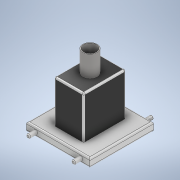
# Autodesk Inventor part: Base Prime
Saved by Autodesk Inventor 2022 (Build 260153000, 153)
## iProperties
Created: 2021-10-29
Part Number: Base Prime
Material: Aluminum 6061
Document SubType Name: Modeling
Designer: Mark Maara
Density: 2.7 g/cm^3
Appearance: Aluminum - Polished
Mass: 6995.86 g
Surface Area: 46826.5 cm^2
Volume: 2591.06 cm^3
Author: Mark Maara
Autodesk Inventor part; units mm, degrees
ref_plane "YZ Plane" through (0, 0, 0) normal (1, 0, 0) x (0, 1, 0)
ref_plane "XZ Plane" through (0, 0, 0) normal (0, 1, 0) x (-1, 0, 0)
ref_plane "XY Plane" through (0, 0, 0) normal (0, 0, 1) x (1, 0, 0)
sketch "Sketch1" plane through (0, 0, 0) normal (0, 1, 0) x (-1, 0, 0)
  circle A0 centre (0, 0) radius 75
  circle A1 centre (0, 0) radius 85
  dimension "d1" = 150
  dimension "d2" = 170
  constraints: 2 centre point, 2 coincident
  measures "d1" diameter of A0
  measures "d2" diameter of A1
extrude "Extrusion1" add sketch "Sketch1" along normal blind 250
sketch "Sketch2" plane through (0, 0, 0) normal (0, -1, 0) x (1, 0, 0)
  line L0 (-175, 250) -> (175, 250)
  line L1 (175, 250) -> (175, -250)
  line L2 (175, -250) -> (-175, -250)
  line L3 (-175, -250) -> (-175, 250)
  line L4 (-175, 250) -> (175, -250) construction
  line L5 (175, 250) -> (-175, -250) construction
  point P0 (0, 0)
  dimension "d5" = 500
  dimension "d6" = 350
  constraints: 12 end point, 2 midpoint, 2 parallel, 1 horizontal, 1 perpendicular
  measures "d5" distance of L0.end L1.end
  measures "d6" distance of L1.end L2.end
extrude "Extrusion2" add sketch "Sketch2" along normal blind 500
sketch "Sketch3" plane through (0, -500, 0) normal (0, -1, 0) x (1, 0, 0)
  line L0 (-375, -375) -> (375, -375)
  line L1 (375, -375) -> (375, 375)
  line L2 (375, 375) -> (-375, 375)
  line L3 (-375, 375) -> (-375, -375)
  line L4 (-375, -375) -> (375, 375) construction
  line L5 (375, -375) -> (-375, 375) construction
  point P0 (0, 0)
  dimension "d9" = 750
  dimension "d10" = 750
  constraints: 12 end point, 2 midpoint, 2 parallel, 1 horizontal, 1 perpendicular
  measures "d9" distance of L1.end L2.end
  measures "d10" distance of L0.end L1.end
extrude "Extrusion3" add sketch "Sketch3" along normal blind 100
fillet "Fillet2" radius 20 8 edges at (-175, -250, -250) (175, -250, -250) (-175, -250, 250) (175, -250, 250) (0, 0, 250) (175, 0, 0) (-175, 0, 0) (0, 0, -250)
fillet "Fillet3" radius 20 8 edges at (0, -600, -375) (0, -500, -375) (-375, -500, 0) (-375, -600, 0) (0, -600, 375) (0, -500, 375) (375, -500, 0) (375, -600, 0)
sketch "Sketch7" plane through (375, -520, -375) normal (0, 0, -1) x (-1, 0, 0)
  line L0 (750, 0) -> (0, 0) projected
  arc A0 (0, -60) -> (20, -80) centre (20, -60) ccw projected
  line L1 (0, 0) -> (0, -60)
  line L2 (109.0667, 0) -> (109.0667, -60)
  line L3 (1, -60) -> (749, -60) projected
  circle A1 centre (109.0667, -30) radius 22.5
  line L4 (375, 0) -> (375, -60)
  circle A2 centre (640.9333, -30) radius 22.5
  point P0 (375, 520)
  dimension "d27" = 45
  constraints: 6 end point, 3 midpoint, 2 centre point, 2 point on line, 2 vertical, 1 symmetric about line, 1 tangent, 1 other
  measures "d27" diameter of A1
extrude "Extrusion7" add sketch "Sketch7" along normal blind 90 contours A1 L2 | L2 A1 | A2
mirror "Mirror4" about plane through (0, 0, 0) normal (0, 0, 1) of "Extrusion7"
fillet "Fillet4" radius 10 4 edges at (-243.4333, -550, 465) (288.4333, -550, 465) (288.4333, -550, -465) (-243.4333, -550, -465)
body "Solid1"
